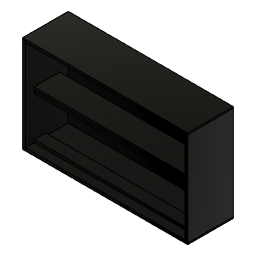
Kosmo Case (Autodesk Fusion 360 design; units mm, degrees)
Autodesk Fusion 360 part; units mm, degrees
sketch "Sketch1" plane through (0, 0, 0) normal (0, 1, 0) x (1, 0, 0)
  line L0 (0, 0) -> (725.424, 0)
  line L1 (725.424, 0) -> (725.424, -200.66)
  line L2 (725.424, -200.66) -> (0, -200.66)
  line L3 (0, -200.66) -> (0, 0)
  line L4 (12.446, -200.66) -> (12.446, -12.446)
  line L5 (712.978, -12.446) -> (712.978, -200.66)
  line L6 (12.446, -12.446) -> (712.978, -12.446)
  dimension "d5" = 725.424
  dimension "d6" = 200.66
  dimension "d31" = 12.446
  dimension "d32" = 12.446
  dimension "d33" = 12.446
  constraint horizontal L0
  constraint vertical L1
  constraint horizontal L2
  constraint vertical L3
  constraint coincident L0.start L3.end
  constraint parallel L0 L6
  constraint parallel L3 L4
  constraint parallel L1 L5
  constraint coincident L2 L4.start
  constraint coincident L2 L5.end
  measures "d5" distance of L0.start L0.end
  measures "d6" distance of L0.start L2.end
  measures "d31" distance of L3 L4
  measures "d32" distance of L0 L6
  measures "d33" distance of L1 L5
extrude "Extrude1" add sketch "Sketch1" along normal blind 6.096 makes body 1
extrude "Extrude2" add sketch "Sketch1" along normal blind 12.192 contours L2 L4 L5 L6 bodies 1
sketch "Sketch2" plane through (0, 6.096, 0) normal (0, 1, 0) x (-1, 0, 0)
  line L0 (-12.446, 200.66) -> (-12.446, 12.446)
  line L1 (-12.446, 12.446) -> (-712.978, 12.446)
  line L2 (-712.978, 12.446) -> (-712.978, 200.66)
  line L3 (-712.978, 200.66) -> (-725.424, 200.66)
  line L4 (-725.424, 200.66) -> (-725.424, 0)
  line L5 (-725.424, 0) -> (0, 0)
  line L6 (0, 0) -> (0, 200.66)
  line L7 (-12.192, 200.66) -> (0, 200.66)
  line L8 (0, 200.66) -> (0, 0)
  line L9 (-12.7, 0) -> (-712.5243, 0)
  line L10 (-712.724, 12.7) -> (-12.7, 12.7)
  line L11 (-6.35, 12.7) -> (-6.35, 0) construction
  line L12 (-6.35, 0) -> (-719.074, 0)
  line L13 (-719.074, 0) -> (-719.074, 12.192)
  line L14 (-719.074, 12.192) -> (-6.35, 12.192)
  line L15 (-6.35, 12.192) -> (-6.35, 0)
  line L16 (-6.096, 12.954) -> (-6.096, 0)
  line L17 (-12.192, 200.66) -> (-12.192, 12.954)
  line L18 (-12.192, 12.954) -> (-6.096, 12.954)
  line L19 (-712.5243, 0) -> (-719.074, 0)
  line L20 (-719.328, 0) -> (-725.2243, 0)
  line L21 (0, 0) -> (-6.096, 0)
  line L22 (-6.35, 0) -> (-12.7, 0)
  line L23 (0, 200.66) -> (-12.446, 200.66)
  dimension "d15" = 200.66
  dimension "d21" = 712.724
  dimension "d22" = 12.192
  dimension "d36" = 12.192
  constraint horizontal L21
  constraint horizontal L7
  constraint vertical L8
  constraint coincident L5.end L6.start
  constraint horizontal L9
  constraint horizontal L10
  constraint horizontal L19
  constraint horizontal L12
  constraint vertical L13
  constraint horizontal L14
  constraint vertical L15
  constraint parallel L8 L17
  constraint parallel L15 L16
  constraint collinear L19 L20
  constraint collinear L21 L22
  measures "d15" distance of L5.end L6.end
  measures "d21" distance of L11.end L12.end
  measures "d22" distance of L11.end L14.end
  measures "d36" distance of L8 L17
copy_body "Body->Comp1" bodies 1 removing the originals makes body 2 in component "Component"
extrude "Extrude3" add sketch "Sketch2" along normal blind 412.242 separate body contours L5 L6 L7 L8 L16 L17 L18 L21 L23 makes body 3
sketch "Sketch5" plane through (12.192, 0, 0) normal (1, 0, 0) x (0, 0, -1)
  line L0 (-200.66, 6.096) -> (-12.954, 6.096)
  line L1 (-12.954, 6.096) -> (-12.954, 418.338)
  line L2 (-12.954, 418.338) -> (-200.66, 418.338)
  line L3 (-200.66, 418.338) -> (-200.66, 6.096)
  line L4 (-200.66, 212.217) -> (-12.954, 212.217)
  line L5 (-150.368, 221.488) -> (-150.368, 203.581)
  line L6 (-62.23, 221.488) -> (-62.23, 203.581)
  line L7 (-147.193, 200.406) -> (-65.405, 200.406)
  line L8 (-147.193, 224.663) -> (-65.405, 224.663)
  arc A0 (-147.193, 224.663) -> (-150.368, 221.488) centre (-147.193, 221.488) ccw
  arc A1 (-150.368, 203.581) -> (-147.193, 200.406) centre (-147.193, 203.581) ccw
  arc A2 (-65.405, 200.406) -> (-62.23, 203.581) centre (-65.405, 203.581) ccw
  arc A3 (-62.23, 221.488) -> (-65.405, 224.663) centre (-65.405, 221.488) ccw
  line L9 (-162.56, 418.338) -> (-162.56, 6.096) construction
  line L10 (-50.038, 418.338) -> (-50.038, 6.096)
  line L11 (-147.193, 224.409) -> (-65.405, 224.409) construction
  line L12 (-147.193, 200.66) -> (-65.405, 200.66) construction
  line L13 (-147.193, 224.409) -> (-162.56, 224.409)
  line L14 (-162.56, 224.409) -> (-162.56, 200.66)
  line L15 (-162.56, 200.66) -> (-147.193, 200.66)
  line L16 (-147.193, 200.66) -> (-147.193, 224.409)
  line L17 (-65.405, 224.409) -> (-50.038, 224.409)
  line L18 (-50.038, 224.409) -> (-50.038, 200.6585)
  line L19 (-50.038, 200.6585) -> (-65.405, 200.6585)
  line L20 (-65.405, 200.6585) -> (-65.405, 224.409)
  dimension "d49" = 50.292
  dimension "d50" = 138.43
  dimension "d51" = 24.892
  dimension "d52" = 3.175
  dimension "d71" = -150.622
  dimension "d72" = 0.254
  constraint midpoint L3 L4.start
  constraint midpoint L1 L4.end
  constraint parallel L4 L8
  constraint parallel L4 L7
  constraint parallel L3 L5
  constraint parallel L3 L6
  constraint tangent L5 A0
  constraint tangent L8 A0
  constraint tangent L5 A1
  constraint tangent L7 A1
  constraint equal A0 A1
  constraint tangent L7 A2
  constraint tangent L6 A2
  constraint equal A0 A2
  constraint tangent L8 A3
  constraint tangent L6 A3
  constraint equal A0 A3
  constraint horizontal L13
  constraint vertical L14
  constraint horizontal L15
  constraint vertical L16
  constraint coincident L9 L14.end
  constraint horizontal L17
  constraint vertical L18
  constraint horizontal L19
  constraint vertical L20
  constraint coincident L10 L18.end
  measures "d49" distance of L3 L5
  measures "d50" distance of L3 L6
  measures "d52" radius of A0
extrude "Extrude4" cut sketch "Sketch5" against normal blind 6.096 contours L4 L6 A2 L19 L20 | L4 L7 A1 A2 L15 L16 L19 L20 | L4 L5 A0 L13 L16 | L4 L5 A1 L15 L16 | L4 L6 A3 L17 L20 | L4 L8 A0 A3 L13 L16 L17 L20 bodies 3
ref_plane "WorkPlane2" through (362.712, 212.217, 100.33) normal (0, 1, 0) x (0, 0, 1)
ref_plane "WorkPlane3" through (362.712, 212.217, 100.33) normal (-1, 0, 0) x (0, 0, 1)
copy_body "CutPasteBodies1" bodies 3 removing the originals makes body 4 in component "Component"
mirror "Mirror1" about plane through (362.712, 212.217, 100.33) normal (0, 1, 0) of bodies 2 makes body 5 in component "Component"
mirror "Mirror2" about plane through (362.712, 212.217, 100.33) normal (-1, 0, 0) of bodies 4 makes body 6 in component "Component"
ref_plane "WorkPlane4" through (362.712, 6.35, 100.33) normal (0, 1, 0) x (0, 0, 1)
sketch "Sketch6" plane through (363.22, 6.35, 100.33) normal (0, 1, 0) x (1, 0, 0)
  line L0 (-356.87, 100.33) -> (356.108, 100.33)
  line L1 (356.108, 100.33) -> (356.108, 88.138)
  line L2 (356.108, 88.138) -> (-356.87, 88.138)
  line L3 (-356.87, 88.138) -> (-356.87, 100.33)
  dimension "d61" = 712.978
  dimension "d62" = 12.192
  constraint horizontal L0
  constraint vertical L1
  constraint horizontal L2
  constraint vertical L3
  measures "d61" distance of L0.start L0.end
  measures "d62" distance of L0.start L2.end
extrude "Extrude5" add sketch "Sketch6" along normal blind 411.734 separate body makes body 7
ref_plane "WorkPlane5" through (6.35, 212.5345, 106.299) normal (1, 0, 0) x (0, 0, -1)
sketch "Sketch7" plane through (6.35, 213.36, 106.045) normal (1, 0, 0) x (0, 0, -1)
  line L0 (-44.323, -9.779) -> (-44.323, 8.128)
  circle A0 centre (-41.148, 8.128) radius 0.001
  line L1 (-41.148, 11.303) -> (40.64, 11.303)
  arc A1 (43.815, 8.128) -> (40.64, 11.303) centre (40.64, 8.128) ccw
  line L2 (43.815, 8.128) -> (43.815, -9.779)
  arc A2 (40.64, -12.954) -> (43.815, -9.779) centre (40.64, -9.779) ccw
  line L3 (-44.323, -9.779) -> (-44.323, 8.128)
  arc A3 (-41.148, 11.303) -> (-44.323, 8.128) centre (-41.148, 8.128) ccw
  line L4 (-41.148, 11.303) -> (40.64, 11.303)
  arc A4 (43.815, 8.128) -> (40.64, 11.303) centre (40.64, 8.128) ccw
  line L5 (43.815, 8.128) -> (43.815, -9.779)
  arc A5 (40.64, -12.954) -> (43.815, -9.779) centre (40.64, -9.779) ccw
  line L6 (40.64, -12.954) -> (-41.148, -12.954)
  arc A6 (-44.323, -9.779) -> (-41.148, -12.954) centre (-41.148, -9.779) ccw
  line L7 (-94.615, -207.264) -> (93.091, -207.264)
  line L8 (93.091, -207.264) -> (93.091, 204.978)
  line L9 (93.091, 204.978) -> (-94.615, 204.978)
  line L10 (-94.615, 204.978) -> (-94.615, -207.264)
  line L11 (-41.148, 11.049) -> (40.64, 11.049)
  line L12 (40.64, -12.7) -> (-41.148, -12.7)
  line L13 (-41.148, 11.049) -> (-41.148, -12.7)
  line L14 (40.64, 11.049) -> (40.64, -12.7)
  line L15 (-41.148, -0.8255) -> (40.64, -0.8255)
  dimension "d66" = 0.254
  dimension "d67" = 0.254
  constraint perpendicular L12 L13
  constraint perpendicular L12 L14
  constraint midpoint L13 L15.start
  constraint midpoint L14 L15.end
ref_plane "WorkPlane6" through (12.446, 315.2775, 125.349) normal (1, 0, 0) x (0, 0, -1)
sketch "Sketch8" plane through (12.446, 316.865, 125.095) normal (1, 0, 0) x (0, 0, -1)
  line L0 (-22.098, -92.456) -> (-37.465, -92.456)
  line L1 (-37.465, -92.456) -> (-37.465, -116.205)
  line L2 (-22.098, -116.205) -> (-22.098, -92.456)
  line L3 (-37.465, -116.205) -> (-22.098, -116.205)
  line L4 (59.69, -116.2065) -> (59.69, -92.456)
  line L5 (59.69, -92.456) -> (75.057, -92.456)
  line L6 (75.057, -92.456) -> (75.057, -116.2065)
  line L7 (75.057, -116.2065) -> (59.69, -116.2065)
  line L8 (112.141, 101.473) -> (-75.565, 101.473)
  line L9 (-37.465, 101.473) -> (-37.465, -310.769)
  line L10 (75.057, 101.473) -> (75.057, -310.769)
  line L11 (-75.565, -104.648) -> (112.141, -104.648)
  line L12 (-75.565, 95.377) -> (112.649, 95.377)
  line L13 (-37.465, 95.377) -> (13.335, 95.377)
  line L14 (13.335, 95.377) -> (13.335, 83.185)
  line L15 (13.335, 83.185) -> (-37.465, 83.185)
  line L16 (-37.465, 83.185) -> (-37.465, 95.377)
  dimension "d83" = 50.8
  dimension "d84" = 12.192
  constraint horizontal L13
  constraint vertical L14
  constraint horizontal L15
  constraint vertical L16
  constraint coincident L12 L13.start
  constraint coincident L9 L13.start
  measures "d83" distance of L13.start L13.end
  measures "d84" distance of L13.start L15.end
extrude "Extrude6" add sketch "Sketch7" along normal blind 712.724 separate body contours L0 L1 A1 L2 A2 L3 A3 L4 A4 L5 A5 L6 A6 | L11 L13 L14 L15 makes body 8
extrude "Extrude7" add sketch "Sketch8" along normal blind 700.532 contours L0 L1 L2 L9 L11 | L4 L5 L6 L10 L11 bodies 8
copy_body "CutPasteBodies2" bodies 7 8 removing the originals makes body 9 makes body 10 in component "Component"
mirror "Mirror3" about plane through (362.712, 212.217, 100.33) normal (0, 1, 0) of bodies 10 makes body 11 in component "Component"
extrude "Extrude1'" add sketch "Sketch8" along normal blind 700.532 separate body contours L9 L12 L13 L14 L15 L16 makes body 12 in component "Component"
mirror "Mirror4" about plane through (362.712, 212.217, 100.33) normal (0, 1, 0) of bodies 12 makes body 13 in component "Component"
component "Component" placed x (1, 0, 0) y (0, 1, 0) z (0, 0, 1) at (0, 0, 0)
equation "Thickness = 0.48 in"
equation "Width = 27.6 in + 2 * Thickness"
equation "Height = 15.75 in + Thickness"
equation "Depth = 7.9 in"
equation "d5 = Width"
equation "d6 = Depth"
equation "d10 = Thickness * 0.5"
equation "d12 = Thickness"
equation "d15 = Depth"
equation "d21 = Width - Thickness - 2 * Tolerance"
equation "d22 = Thickness"
equation "d23 = Height"
equation "Inset = 1.5 in"
equation "Tolerance = 0.01 in"
equation "d31 = Thickness + Tolerance"
equation "d32 = Thickness + Tolerance"
equation "d33 = Thickness + Tolerance"
equation "d36 = Thickness"
equation "d47 = -Thickness / 2"
equation "d49 = Inset + Thickness"
equation "d50 = Inset + Depth / 2"
equation "d51 = ( Thickness + Tolerance ) * 2"
equation "d54 = Height / 2"
equation "d55 = -Width / 2"
equation "d60 = Tolerance"
equation "d61 = Width - Thickness - Tolerance"
equation "d62 = Thickness"
equation "d63 = Height - 2 * Tolerance"
equation "d65 = Tolerance"
equation "d66 = Tolerance"
equation "d67 = Tolerance"
equation "d68 = Width - Thickness - 2 * Tolerance"
equation "d70 = -Inset"
equation "d71 = -Inset - Depth / 2 - Thickness"
equation "d72 = Tolerance"
equation "d73 = -Tolerance"
equation "d74 = Width - 2 * Thickness - 2 * Tolerance"
equation "d78 = Tolerance"
equation "d81 = Width - ( 2 * Thickness ) - 2 * Tolerance"
equation "d84 = Thickness"
named bodies: "Bottom", "Left Side", "Top", "Right Side", "Back", "Shelf", "Top Shelf", "Bottom Shelf", "Top Rail", "Bottom Rail"
